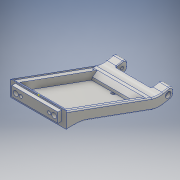
# Autodesk Inventor part: primoblocco
Saved by Autodesk Inventor 2016 (Build 200138000, 138)
## iProperties
Created: 2017-09-06
Part Number: primoblocco
Material: Aluminum 6061
Document SubType Name: Modeling
Designer: Davide
Density: 2.7 g/cm^3
Appearance: Aluminum - Flat
Mass: 290.704 g
Surface Area: 358.316 cm^2
Volume: 107.668 cm^3
Author: Davide
Autodesk Inventor part; units mm, degrees
ref_plane "YZ Plane" through (0, 0, 0) normal (1, 0, 0) x (0, 1, 0)
ref_plane "XZ Plane" through (0, 0, 0) normal (0, 1, 0) x (-1, 0, 0)
ref_plane "XY Plane" through (0, 0, 0) normal (0, 0, 1) x (1, 0, 0)
sketch "Sketch1" plane through (0, 0, 0) normal (1, 0, 0) x (0, 1, 0)
  line L0 (28.8907, -25.5154) -> (119.7394, -58.5816)
  line L1 (135.2094, -59.935) -> (150, -57.3271)
  line L2 (0, 0) -> (0, -22.5)
  line L3 (150, -57.3271) -> (150, -42.3271)
  line L4 (150, -42.3271) -> (135.2094, -44.935)
  line L5 (0, 0) -> (119.7394, -43.5816)
  arc A0 (119.7394, -58.5816) -> (135.2094, -59.935) centre (130, -30.3908) ccw
  arc A1 (119.7394, -43.5816) -> (135.2094, -44.935) centre (130, -15.3908) ccw
  line L6 (0, -22.5) -> (11.7897, -22.5)
  arc A2 (28.8907, -25.5154) -> (11.7897, -22.5) centre (11.7897, -72.5) ccw
  dimension "d0" = 70
  dimension "d1" = 150
  dimension "d2" = 150
  dimension "d4" = 30
  dimension "d5" = 50
  dimension "d6" = 15
  dimension "d7" = 130
  dimension "d8" = 130
  dimension "d9" = 22.5
  constraints: 14 end point, 6 point on circle, 6 tangent, 3 centre point, 2 parallel, 2 vertical, 1 coincident, 1 equal radius, 1 horizontal
  measures "d0" angle of L2 L0
  measures "d1" angle of L0 L1
  measures "d2" distance between parallel lines of L2 L3
  measures "d4" radius of A0
  measures "d5" radius of A2
  measures "d6" distance of L1.end L3.end
  measures "d7" horizontal distance of point (0, 0) A0.centre
  measures "d8" horizontal distance of point (0, 0) A1.centre
  measures "d9" distance of L2.start L2.end
extrude "Extrusion1" add sketch "Sketch1" along normal mid plane 80
fillet "Fillet1" radius 5 2 edges at (0, 150, -42.3271) (0, 150, -57.3271)
sketch "Sketch2" plane through (40, 0, 0) normal (1, 0, 0) x (0, 0, -1)
  arc A0 (58.0556, 145.8682) -> (53.1316, 150) centre (53.1316, 145) ccw projected
  line L0 (53.1316, 150) -> (48.2858, 150) projected
  arc A1 (48.2858, 150) -> (43.3618, 144.1318) centre (48.2858, 145) ccw projected
  line L1 (43.3618, 144.1318) -> (44.935, 135.2094) projected
  arc A2 (43.5816, 119.7394) -> (44.935, 135.2094) centre (15.3908, 130) ccw projected
  line L2 (43.5816, 119.7394) -> (0, 0) projected
  line L3 (0, 0) -> (22.5, 0) projected
  line L4 (22.5, 0) -> (22.5, 11.7897) projected
  arc A3 (25.5154, 28.8907) -> (22.5, 11.7897) centre (72.5, 11.7897) ccw projected
  line L5 (25.5154, 28.8907) -> (58.5816, 119.7394) projected
  arc A4 (58.5816, 119.7394) -> (59.935, 135.2094) centre (30.3908, 130) ccw projected
  line L6 (59.935, 135.2094) -> (58.0556, 145.8682) projected
  circle A5 centre (51.1294, 142.6139) radius 7.3861 construction
  circle A6 centre (51.1294, 142.6139) radius 2
  circle A7 centre (51.1294, 142.6139) radius 4
  dimension "d13" = 4
  dimension "d113" = 8
  constraints: 3 centre point, 3 tangent, 2 coincident
  measures "d13" diameter of A6
  measures "d113" diameter of A7
extrude "Extrusion2" cut sketch "Sketch2" against normal through all contours A6
sketch "Sketch3" plane through (-40, 150, -48.2858) normal (0, 1, 0) x (1, 0, 0)
  line L0 (40, -48.2858) -> (40, 25.6638) construction
  line L1 (15, -12.7465) -> (65, -12.7465)
  line L2 (65, -12.7465) -> (65, 27.1757)
  line L3 (65, 27.1757) -> (15, 27.1757)
  line L4 (15, 27.1757) -> (15, -12.7465)
  point P0 (40, -12.7465)
  dimension "d16" = 39.9222
  dimension "d17" = 50
  constraints: 10 end point, 2 parallel, 1 horizontal, 1 midpoint, 1 perpendicular, 1 point on line, 1 vertical
  measures "d16" distance of L3.end L1.start
  measures "d17" distance of L2.end L3.end
extrude "Extrusion3" cut sketch "Sketch3" against normal blind 16
fillet "Fillet2" radius 1.5 2 edges at (-25, 134, -52.6229) (25, 134, -52.6229)
fillet "Fillet3" radius 1.5 22 edges at (40, 150, -50.7087) (40, 148.8302, -56.3455) (40, 140.5388, -58.9953) (40, 127.3853, -60.2766) (40, 74.3151, -42.0485) (40, 20.4721, -23.2596) (40, 5.8949, -22.5) (40, 139.6706, -44.1484) (40, 127.3853, -45.2766) (40, 59.8697, -21.7908) (40, 148.2139, -44.4556) (-40, 127.3853, -45.2766) (-40, 139.6706, -44.1484) (-40, 148.2139, -44.4556) (-40, 150, -50.7087) (-40, 148.8302, -56.3455) (-40, 140.5388, -58.9953) (-40, 127.3853, -60.2766) (-40, 74.3151, -42.0485) (-40, 20.4721, -23.2596) (-40, 5.8949, -22.5) (-40, 59.8697, -21.7908)
fillet "Fillet4" radius 1 20 edges at (-25, 148.2139, -44.4556) (-25, 150, -50.7087) (-25, 148.8302, -56.3455) (-25, 140.6841, -58.9697) (-24.9929, 135.354, -59.9095) (-24.3984, 134.2988, -60.0812) (0, 134, -60.1229) (24.3984, 134.2988, -60.0812) (24.9929, 135.354, -59.9095) (25, 140.6841, -58.9697) (25, 148.8302, -56.3455) (25, 150, -50.7087) (25, 148.2139, -44.4556) (25, 139.8159, -44.1228) (24.9929, 135.354, -44.9095) (24.3975, 134.2981, -45.0813) (0, 134, -45.1229) (-24.3981, 134.2985, -45.0812) (-24.9929, 135.354, -44.9095) (-25, 139.8159, -44.1228)
sketch "Sketch4" plane through (-38.5, 0, -22.5) normal (0, -1, 0) x (1, 0, 0)
  line L0 (38.5, 22.5) -> (38.5, 0) construction
  arc A0 (-1.5, 1.5) -> (0, 0) centre (0, 1.5) ccw projected
  line L1 (77, 0) -> (0, 0) projected
  arc A1 (77, 0) -> (78.5, 1.5) centre (77, 1.5) ccw projected
  line L2 (78.5, 20.9037) -> (78.5, 1.5) projected
  ellipse E0 centre (77, 20.9037) end of major axis (77, 22.5) minor radius 1.5 (78.5, 20.9037) -> (77, 22.5) ccw projected
  line L3 (77, 22.5) -> (0, 22.5) projected
  ellipse E1 centre (0, 20.9037) end of major axis (0, 22.5) minor radius 1.5 (0, 22.5) -> (-1.5, 20.9037) ccw projected
  line L4 (-1.5, 1.5) -> (-1.5, 20.9037) projected
  line L5 (70.9, 20.4) -> (6.1, 20.4)
  line L6 (6.1, 20.4) -> (6.1, 6.6)
  line L7 (6.1, 6.6) -> (70.9, 6.6)
  line L8 (70.9, 6.6) -> (70.9, 20.4)
  point P0 (38.5, 20.4)
  point P1 (70.9, 13.5)
  dimension "d23" = 13.8
  dimension "d24" = 64.8
  dimension "d108" = 9
  constraints: 10 end point, 3 midpoint, 2 parallel, 1 horizontal, 1 perpendicular, 1 point on line, 1 vertical, 2 other
  measures "d23" distance of L5.end L6.end
  measures "d24" distance of L5.start L5.end
  measures "d108" vertical distance of L0.start point (70.9, 13.5)
extrude "Extrusion4" add sketch "Sketch4" along normal blind 5 contours L8 L7 L6 L5
sketch "Sketch5" plane through (-38.5, -5, -22.5) normal (0, -1, 0) x (1, 0, 0)
  circle A0 centre (18.5, 13.5) radius 2.25
  line L0 (6.1, 20.4) -> (6.1, 6.6) projected
  line L1 (6.1, 13.5) -> (70.9, 13.5) construction
  line L2 (70.9, 6.6) -> (70.9, 20.4) projected
  line L3 (38.5, 22.5) -> (38.5, 1.6044) construction
  circle A1 centre (58.5, 13.5) radius 2.25
  dimension "d28" = 40
  dimension "d29" = 4.5
  constraints: 4 end point, 2 centre point, 2 midpoint, 1 point on line, 1 symmetric about line, 1 vertical, 1 other
  measures "d28" distance of A1.centre A0.centre
  measures "d29" diameter of A0
extrude "Extrusion5" cut sketch "Sketch5" against normal blind 20
sketch "Sketch8" plane through (-38.5, 0, 0) normal (0, 0.3420201, 0.9396926) x (1, 0, 0)
  point P0 (38.5, 0)
sketch "Sketch9" plane through (-38.5, 0, 0) normal (0, 0.3420201, 0.9396926) x (1, 0, 0)
  line L0 (0, 0) -> (0, 127.424) projected
  line L1 (77, 0) -> (0, 0) projected
  line L2 (77, 127.424) -> (77, 0) projected
  line L3 (77, 127.424) -> (0, 127.424) projected
  line L4 (0, 127.424) -> (77, 127.424)
  line L5 (77, 127.424) -> (77, 1.5)
  line L6 (77, 1.5) -> (0, 1.5)
  line L7 (0, 1.5) -> (0, 127.424)
  line L8 (0, 123.424) -> (77, 123.424)
  point P0 (38.5, 0)
  dimension "d74" = 1.5
  dimension "d96" = 4
  constraints: 10 end point, 3 point on line, 2 parallel, 2 perpendicular, 1 horizontal
  measures "d74" distance between parallel lines of L1 L6
  measures "d96" distance between parallel lines of L8 L3
ref_plane "Work Plane1" through (-38.5, -0.513, -1.4095) normal (0, 0.3420201, 0.9396926) x (1, 0, 0)
ref_plane "Work Plane2" through (-38.5, -0.513, -1.4095) normal (0, 0.3420201, 0.9396926) x (1, 0, 0)
sketch "Sketch12" plane through (-38.5, -5, -22.5) normal (0, -1, 0) x (1, 0, 0)
  circle A0 centre (18.5, 13.5) radius 2.25 projected
  circle A1 centre (58.5, 13.5) radius 2.25 projected
  line L0 (70.9, 20.4) -> (6.1, 20.4) projected
  line L1 (6.1, 20.4) -> (6.1, 6.6) projected
  line L2 (6.1, 6.6) -> (70.9, 6.6) projected
  line L3 (70.9, 6.6) -> (70.9, 20.4) projected
  circle A2 centre (65.5, 13.5) radius 3.5
  circle A3 centre (11.5, 13.5) radius 3.5
  line L4 (6.1, 13.5) -> (70.9, 13.5) construction
  line L5 (38.5, 13.5) -> (38.5, 9.2182) construction
  point P0 (38.5, 22.5)
  dimension "d68" = 7
  dimension "d69" = 7
  dimension "d70" = 27
  dimension "d71" = 27
  constraints: 4 end point, 3 midpoint, 2 centre point, 2 point on line, 1 horizontal, 1 vertical
  measures "d68" diameter of A2
  measures "d69" diameter of A3
  measures "d70" distance from line of A2.centre L5
  measures "d71" distance from line of L5 A3.centre
extrude "Extrusion12" cut sketch "Sketch12" against normal up to next contours A2 | A3
sketch "Sketch11" plane through (-38.5, -0.513, -1.4095) normal (0, 0.3420201, 0.9396926) x (1, 0, 0)
  line L0 (38.5, 0) -> (38.5, 170.5031) construction
  line L1 (6, 10.546) -> (71, 10.546)
  line L2 (71, 10.546) -> (71, 118.546)
  line L3 (71, 118.546) -> (6, 118.546)
  line L4 (6, 118.546) -> (6, 10.546)
  line L5 (77, 0.546) -> (0, 0.546) projected
  point P0 (38.5, 10.546)
  dimension "d65" = 0
  dimension "d62" = 10
  dimension "d63" = 65
  dimension "d64" = 108
  constraints: 10 end point, 5 horizontal, 5 vertical, 2 parallel, 1 midpoint, 1 perpendicular, 1 point on line, 16 other
  measures "d62" distance between parallel lines of L5 L1
  measures "d63" distance between parallel lines of L2 L4
  measures "d64" distance between parallel lines of L1 L3
extrude "Extrusion11" cut sketch "Sketch11" against normal blind 10.4
ref_plane "Work Plane3" through (-38.5, -0.513, -1.4095) normal (0, 0.3420201, 0.9396926) x (1, 0, 0)
sketch "Sketch13" plane through (-38.5, -0.513, -1.4095) normal (0, 0.3420201, 0.9396926) x (1, 0, 0)
  line L0 (0, 1.5) -> (0, 127.424) projected
  line L1 (77, 1.5) -> (0, 1.5) projected
  line L2 (77, 127.424) -> (0, 127.424) projected
  line L3 (77, 127.424) -> (77, 1.5) projected
  point P0 (38.5, 0)
  point P1 (3, 120.424)
  point P2 (74, 120.424)
  point P3 (74, 4.5)
  point P4 (3, 4.5)
  dimension "d77" = 3
  dimension "d78" = 3
  dimension "d79" = 7
  dimension "d80" = 3
  dimension "d81" = 3
  dimension "d82" = 3
  dimension "d83" = 3
  dimension "d84" = 7
  measures "d77" distance from line of L0 point (3, 4.5)
  measures "d78" distance from line of L1 point (3, 4.5)
  measures "d79" distance from line of point (3, 120.424) L2
  measures "d80" distance from line of L3 point (74, 120.424)
  measures "d81" distance from line of L3 point (74, 4.5)
  measures "d82" distance from line of L1 point (74, 4.5)
  measures "d83" distance from line of L0 point (3, 120.424)
  measures "d84" distance from line of L2 point (74, 120.424)
hole "Hole1" at (-35.5, 112.6485, -42.597) at (35.5, 112.6485, -42.597) at (35.5, 3.7156, -2.9486) at (-35.5, 3.7156, -2.9486) direction (0, -0.3420201, -0.9396926) diameter 1.8 depth 4 tip angle 118
sketch "Sketch14" plane through (-38.5, -4.07, -11.1823) normal (0, 0.3420201, 0.9396926) x (1, 0, 0)
  point P0 (38.5, 0)
sketch "Sketch15" plane through (-38.5, -4.07, -11.1823) normal (0, 0.3420201, 0.9396926) x (1, 0, 0)
  line L0 (71, 118.546) -> (71, 10.546) projected
  line L1 (6, 118.546) -> (71, 118.546) projected
  line L2 (6, 10.546) -> (6, 118.546) projected
  line L3 (71, 10.546) -> (6, 10.546) projected
  line L4 (38.5, 118.546) -> (38.5, 72.8509) construction
  circle A0 centre (38.5, 115.546) radius 2.5
  line L5 (9, 120.546) -> (71, 120.546) projected
  point P0 (38.5, 0)
  point P1 (9, 118.546)
  dimension "d92" = 5
  dimension "d93" = 5
  constraints: 2 end point, 1 centre point, 1 midpoint, 1 point on line, 1 vertical
  measures "d92" diameter of A0
  measures "d93" distance from line of L5 A0.centre
extrude "Extrusion14" cut sketch "Sketch15" against normal through all contours A0
extrude "Extrusion15" cut sketch "Sketch9" against normal blind 1.6 contours L0 L8 L2 L6
sketch "Sketch16" plane through (-38.5, 1.4095, -0.513) normal (1, 0, 0) x (0, -0.3420201, -0.9396926)
  line L0 (0, 121.924) -> (1.6, 121.924) projected
  line L1 (1.5, 125.924) -> (0, 125.924) projected
  line L2 (0, 121.924) -> (1.6, 121.924)
  line L3 (0, 125.924) -> (1.6, 121.924)
  line L4 (0, 121.924) -> (0, 125.924) projected
  line L5 (0, 121.924) -> (0, 125.924)
  point P0 (0, -1.5)
  constraints: 6 end point, 1 horizontal, 1 vertical
extrude "Extrusion16" cut sketch "Sketch16" along normal blind 77
sketch "Sketch17" plane through (-32.5, 9.3627, -5.1104) normal (1, 0, 0) x (0, -0.3420201, -0.9396926)
  line L0 (-0.1, -10) -> (-0.1, 116.878) projected
  line L1 (0, 108) -> (10.3, 108) projected
  line L2 (0, 112.878) -> (-1.6, 116.878) projected
  line L3 (0, 112.878) -> (0, 108)
  line L4 (7, 108) -> (0, 112.878)
  point P0 (-1.6, -10.546)
  point P1 (-0.1, 116.878)
  constraints: 4 end point, 1 vertical, 1 other
extrude "Extrusion18" cut sketch "Sketch17" along normal blind 65
sketch "Sketch18" plane through (32.5, 5.8399, -14.7893) normal (-1, 0, 0) x (0, 0.3420201, 0.9396926)
  line L0 (0, 0) -> (10.4, -3.7853)
  line L1 (10.4, -10) -> (10.4, 116.878) projected
  line L2 (-7.8335, -3.3635) -> (10.4, -10) projected
  line L3 (10.4, -3.7853) -> (10.4, 0)
  line L4 (10.4, 0) -> (0, 0)
  point P0 (11.9, -10.546)
  point P1 (10.3, 0)
  point P2 (10.4, 116.878)
  constraints: 6 end point, 1 horizontal, 1 parallel, 4 other
extrude "Extrusion20" cut sketch "Sketch18" along normal up to surface (65 mm away)
extrude "Extrusion21" cut sketch "Sketch2" against normal blind 4 contours A7
mirror "Mirror1" about plane through (0, 0, 0) normal (1, 0, 0) of "Extrusion21"
equation "\"d8\" = d7"
equation "\"d9\" = 1.5 * d6"
equation "\"d69\" = d68"
equation "\"d71\" = d70"
body "Solid1"
